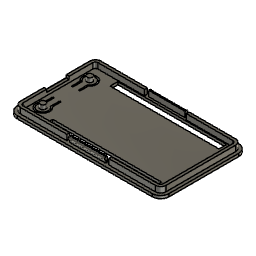
esp32-case (Autodesk Fusion 360 design; units mm, degrees)
Autodesk Fusion 360 part; units mm, degrees
sketch "Sketch3" plane through (0, 0, 0) normal (0, 0, 1) x (1, 0, 0)
  line L0 (0, 13.1652) -> (0, -15.9653) construction
  line L1 (-26.7542, 0) -> (30.5292, 0) construction
  line L2 (23.4, 11.7) -> (-23.4, 11.7)
  line L3 (-23.4, 11.7) -> (-23.4, -11.7)
  line L4 (-23.4, -11.7) -> (23.4, -11.7)
  line L5 (23.4, -11.7) -> (23.4, 11.7)
  line L6 (23.4, 11.7) -> (-23.4, -11.7) construction
  line L7 (-23.4, 11.7) -> (23.4, -11.7) construction
  line L8 (24.2, 14.5) -> (-24.2, 14.5)
  line L9 (-26.2, 12.5) -> (-26.2, -12.5)
  line L10 (-24.2, -14.5) -> (24.2, -14.5)
  line L11 (26.2, -12.5) -> (26.2, 12.5)
  line L12 (26.2, 14.5) -> (-26.2, -14.5) construction
  line L13 (-26.2, 14.5) -> (26.2, -14.5) construction
  arc A0 (-24.2, 14.5) -> (-26.2, 12.5) centre (-24.2, 12.5) ccw
  arc A1 (-26.2, -12.5) -> (-24.2, -14.5) centre (-24.2, -12.5) ccw
  arc A2 (24.2, -14.5) -> (26.2, -12.5) centre (24.2, -12.5) ccw
  arc A3 (26.2, 12.5) -> (24.2, 14.5) centre (24.2, 12.5) ccw
  circle A4 centre (23.4, 11.7) radius 1.1
  line L14 (23.4, 10.6) -> (26.2, 10.6)
  line L15 (22.3, 11.7) -> (22.3, 14.5)
  circle A5 centre (-23.4, 11.7) radius 1.1
  line L16 (-22.3, 11.7) -> (-22.3, 14.5)
  line L17 (-23.4, 10.6) -> (-26.2, 10.6)
  line L18 (23.4, -10.6) -> (26.2, -10.6)
  line L19 (22.3, -11.7) -> (22.3, -14.5)
  circle A6 centre (23.4, -11.7) radius 1.1
  line L20 (-22.3, -11.7) -> (-22.3, -14.5)
  circle A7 centre (-23.4, -11.7) radius 1.1
  line L21 (-23.4, -10.6) -> (-26.2, -10.6)
  line L22 (-24.2, -15.5) -> (24.2, -15.5)
  arc A8 (24.2, -15.5) -> (27.2, -12.5) centre (24.2, -12.5) ccw
  line L23 (27.2, -12.5) -> (27.2, 12.5)
  arc A9 (27.2, 12.5) -> (24.2, 15.5) centre (24.2, 12.5) ccw
  line L24 (24.2, 15.5) -> (-24.2, 15.5)
  arc A10 (-24.2, 15.5) -> (-27.2, 12.5) centre (-24.2, 12.5) ccw
  line L25 (-27.2, 12.5) -> (-27.2, -12.5)
  arc A11 (-27.2, -12.5) -> (-24.2, -15.5) centre (-24.2, -12.5) ccw
  line L26 (-16.7, 14.5) -> (-16.7, 11.7)
  line L27 (-16.7, -14.5) -> (-16.7, -11.7)
  line L28 (-26.2, 0) -> (-27.2, 0)
  line L29 (-27.2, 0) -> (-27.2, 4)
  line L30 (-27.2, 4) -> (-26.2, 4)
  line L31 (-26.2, 4) -> (-26.2, 0)
  line L32 (-27.2, 0) -> (-27.2, -4)
  line L33 (-27.2, -4) -> (-26.2, -4)
  line L34 (-26.2, 0) -> (-27.2, 0)
  dimension "d52" = 46.8
  dimension "d53" = 23.4
  dimension "d54" = 29
  dimension "d55" = 52.4
  dimension "d56" = 2
  dimension "d57" = 2.2
  dimension "d59" = 1
  dimension "d61" = 39
  dimension "d78" = 4
  dimension "d79" = 1
  constraint vertical L0
  constraint horizontal L1
  constraint horizontal L2
  constraint perpendicular L2 L3
  constraint parallel L2 L4
  constraint parallel L3 L5
  constraint coincident L6 origin
  constraint coincident L7 origin
  constraint horizontal L8
  constraint perpendicular L8 L9
  constraint parallel L8 L10
  constraint parallel L9 L11
  constraint coincident L12 origin
  constraint coincident L13 origin
  constraint coincident L13.start L8
  constraint coincident L13.start L9
  constraint tangent L8 A0
  constraint tangent L9 A0
  constraint coincident L12.end L9
  constraint coincident L12.end L10
  constraint tangent L9 A1
  constraint tangent L10 A1
  constraint equal A0 A1
  constraint coincident L13.end L10
  constraint coincident L13.end L11
  constraint tangent L10 A2
  constraint tangent L11 A2
  constraint equal A0 A2
  constraint coincident L12.start L11
  constraint coincident L12.start L8
  constraint tangent L11 A3
  constraint tangent L8 A3
  constraint equal A0 A3
  constraint coincident L2.start L5.end
  constraint coincident A4 L14.start
  constraint coincident L5 L14.start
  constraint coincident L11 L14.end
  constraint tangent A4 L14
  constraint coincident A4 L15.start
  constraint coincident L2 L15.start
  constraint coincident L8 L15.end
  constraint tangent A4 L15
  constraint coincident L1 origin
  constraint coincident L0 origin
  constraint symmetric L0 A4 A5
  constraint symmetric L0 L14.start L17.start
  constraint symmetric L0 L14.end L17.end
  constraint symmetric L0 L15.start L16.start
  constraint symmetric L0 L15.end L16.end
  constraint symmetric L1 A4 A6
  constraint symmetric L1 L14.start L18.start
  constraint symmetric L1 L14.end L18.end
  constraint symmetric L1 L15.start L19.start
  constraint symmetric L1 L15.end L19.end
  constraint symmetric L1 A5 A7
  constraint symmetric L1 L16.start L20.start
  constraint symmetric L1 L16.end L20.end
  constraint symmetric L1 L17.start L21.start
  constraint symmetric L1 L17.end L21.end
  constraint coincident L8 L26.start
  constraint coincident L2 L26.end
  constraint perpendicular L2 L26
  constraint symmetric L1 L26.start L27.start
  constraint symmetric L1 L26.end L27.end
  constraint horizontal L28
  constraint vertical L29
  constraint horizontal L30
  constraint vertical L31
  constraint midpoint L9 L28.start
  constraint symmetric L1 L28.start L31.end
  constraint symmetric L1 L28.end L29.start
  constraint symmetric L1 L29.end L32.end
  constraint symmetric L1 L30.end L33.end
  measures "d52" distance of L3.end L4.end
  measures "d53" distance of L2.end L3.end
  measures "d54" distance of L13.start L12.end
  measures "d55" distance of L13.end L9
  measures "d56" radius of A0
  measures "d57" diameter of A4
  measures "d61" distance of L15 L26
  measures "d78" distance of L28.start L30.end
  measures "d79" distance of L29 L31
extrude "Extrude14" add sketch "Sketch3" along normal blind 1 contours L2 L5 A4 | L2 L5 A4 | L2 L3 L4 L5 A4 A5 A6 A7 | L8 L11 A3 A4 L14 L15 | L5 L11 L14 L18 | L2 L8 L16 L26 | L8 L9 L10 L11 A0 A1 A2 A3 L22 A8 L23 A9 L24 A10 L25 A11 L30 L33 | L4 L5 A6 | L10 L11 A2 L18 L19 A6 | L4 L5 A6 | L2 L3 A5 | L2 L3 A5 | L8 L9 A0 A5 L16 L17 | L3 L9 L17 L21 L31 | L4 L10 L20 L27 | L3 L4 A7 | L3 L4 A7 | L9 L10 A1 L20 A7 L21 | L9 L25 L28 L29 L30 L31 L34 | L9 L25 L28 L32 L33 L34 makes body 1
extrude "Extrude20" add sketch "Sketch3" along normal blind 13.7 contours L8 L9 L10 L11 A0 A1 A2 A3 L22 A8 L23 A9 L24 A10 L25 A11 L30 L33 bodies 1
extrude "Extrude17" add sketch "Sketch3" along normal blind 8.5 contours L8 L11 A3 A4 L14 L15 | L10 L11 A2 L18 L19 A6 | L8 L9 A0 A5 L16 L17 | L9 L10 A1 L20 A7 L21 bodies 1
extrude "Extrude19" add sketch "Sketch3" along normal blind 10 contours L2 L5 A4 | L2 L5 A4 | L4 L5 A6 | L4 L5 A6 | L2 L3 A5 | L2 L3 A5 | L3 L4 A7 | L3 L4 A7 | L9 L25 L28 L29 L30 L31 L34 | L9 L25 L28 L32 L33 L34 bodies 1
chamfer "Chamfer4" distance 1.3 angle 45 2 edges at (-26.7, 4, 10) (-26.7, -4, 10) on bodies 1
sketch "Sketch2" plane through (0, 0, 0) normal (1, 0, 0) x (0, 1, 0)
  line L0 (0, 15.9882) -> (0, -1.7691) construction
  line L1 (14.5, 13.7) -> (15, 13.7)
  line L2 (15, 13.7) -> (15, 11.7)
  line L3 (15, 11.7) -> (14.5, 11.7)
  line L4 (14.5, 11.7) -> (14.5, 13.7)
  line L5 (-12.5, 0) -> (12.5, 0)
  circle A0 centre (15.0004, 13.2) radius 0.5
  circle A1 centre (-15.0004, 13.2) radius 0.5
  line L6 (-14.5, 13.7) -> (-15, 13.7)
  line L7 (-14.5, 11.7) -> (-14.5, 13.7)
  line L8 (-15, 11.7) -> (-14.5, 11.7)
  line L9 (-15, 13.7) -> (-15, 11.7)
  dimension "d26" = 0.5
  dimension "d27" = 2
  dimension "d28" = 14.5
  dimension "d73" = 1
  constraint vertical L0
  constraint horizontal L1
  constraint vertical L2
  constraint horizontal L3
  constraint vertical L4
  constraint coincident origin L0
  constraint coincident L1.end A0
  constraint symmetric L0 L1.start L6.start
  constraint symmetric L0 L1.end L6.end
  constraint symmetric L0 L2.end L8.start
  constraint symmetric L0 L3.end L7.start
  constraint symmetric L0 A0 A1
  measures "d26" distance of L1.start L1.end
  measures "d27" distance of L1.start L3.end
  measures "d28" distance of L0 L4
  measures "d73" diameter of A0
extrude "Extrude18" cut sketch "Sketch2" along normal mid plane 14 contours L1 L4 A0 | L2 L3 L4 A0 | A1 L7 L8 L9 | A1 L6 L7 bodies 1
sketch "Sketch4" plane through (0, 0, 0) normal (0, 0, 1) x (1, 0, 0)
  line L0 (0, 24.6712) -> (0, -25.9096) construction
  line L1 (-37.8993, 0) -> (40.7367, 0) construction
  line L2 (-24.2, -14.5) -> (24.2, -14.5)
  line L3 (26.2, -12.5) -> (26.2, 12.5)
  line L4 (24.2, 14.5) -> (-24.2, 14.5)
  line L5 (-26.2, 12.5) -> (-26.2, -12.5)
  line L6 (-26.2, -14.5) -> (26.2, 14.5) construction
  line L7 (26.2, -14.5) -> (-26.2, 14.5) construction
  arc A0 (-24.2, 14.5) -> (-26.2, 12.5) centre (-24.2, 12.5) ccw
  arc A1 (-26.2, -12.5) -> (-24.2, -14.5) centre (-24.2, -12.5) ccw
  arc A2 (24.2, -14.5) -> (26.2, -12.5) centre (24.2, -12.5) ccw
  arc A3 (26.2, 12.5) -> (24.2, 14.5) centre (24.2, 12.5) ccw
  line L8 (-24.2, -15.5) -> (24.2, -15.5)
  arc A4 (24.2, -15.5) -> (27.2, -12.5) centre (24.2, -12.5) ccw
  line L9 (27.2, -12.5) -> (27.2, 12.5)
  arc A5 (27.2, 12.5) -> (24.2, 15.5) centre (24.2, 12.5) ccw
  line L10 (24.2, 15.5) -> (-24.2, 15.5)
  arc A6 (-24.2, 15.5) -> (-27.2, 12.5) centre (-24.2, 12.5) ccw
  line L11 (-27.2, 12.5) -> (-27.2, -12.5)
  arc A7 (-27.2, -12.5) -> (-24.2, -15.5) centre (-24.2, -12.5) ccw
  line L12 (-26.1, 12.5) -> (-26.1, -12.5)
  arc A8 (-26.1, -12.5) -> (-24.2, -14.4) centre (-24.2, -12.5) ccw
  line L13 (-24.2, -14.4) -> (24.2, -14.4)
  arc A9 (24.2, -14.4) -> (26.1, -12.5) centre (24.2, -12.5) ccw
  line L14 (26.1, -12.5) -> (26.1, 12.5)
  arc A10 (26.1, 12.5) -> (24.2, 14.4) centre (24.2, 12.5) ccw
  line L15 (24.2, 14.4) -> (-24.2, 14.4)
  arc A11 (-24.2, 14.4) -> (-26.1, 12.5) centre (-24.2, 12.5) ccw
  line L16 (-24.2, -13.4) -> (24.2, -13.4)
  arc A12 (24.2, -13.4) -> (25.1, -12.5) centre (24.2, -12.5) ccw
  line L17 (25.1, -12.5) -> (25.1, 12.5)
  arc A13 (25.1, 12.5) -> (24.2, 13.4) centre (24.2, 12.5) ccw
  line L18 (24.2, 13.4) -> (-24.2, 13.4)
  arc A14 (-24.2, 13.4) -> (-25.1, 12.5) centre (-24.2, 12.5) ccw
  line L19 (-25.1, 12.5) -> (-25.1, -12.5)
  arc A15 (-25.1, -12.5) -> (-24.2, -13.4) centre (-24.2, -12.5) ccw
  line L20 (-22.1, 14.4) -> (-26.1, 14.4) construction
  line L21 (-26.1, 14.4) -> (-26.1, 8.4) construction
  line L22 (-26.1, 8.4) -> (-22.1, 8.4) construction
  line L23 (-22.1, 8.4) -> (-22.1, 14.4) construction
  circle A16 centre (-22.1, 8.4) radius 1
  circle A17 centre (-22.1, 8.4) radius 2
  circle A18 centre (-22.1, 8.4) radius 2.5
  line L24 (-23.6, 3.4) -> (-20.6, 3.4)
  line L25 (-20.6, 3.4) -> (-20.6, 13.4)
  line L26 (-20.6, 13.4) -> (-23.6, 13.4)
  line L27 (-23.6, 13.4) -> (-23.6, 3.4)
  line L28 (-23.6, 3.4) -> (-20.6, 13.4) construction
  line L29 (-20.6, 3.4) -> (-23.6, 13.4) construction
  line L30 (-23.1, 13.4) -> (-21.1, 13.4)
  line L31 (-21.1, 13.4) -> (-21.1, 3.4)
  line L32 (-21.1, 3.4) -> (-23.1, 3.4)
  line L33 (-23.1, 3.4) -> (-23.1, 13.4)
  line L34 (-23.1, 13.4) -> (-21.1, 3.4) construction
  line L35 (-21.1, 13.4) -> (-23.1, 3.4) construction
  circle A19 centre (-22.1, -8.4) radius 1
  circle A20 centre (-22.1, -8.4) radius 2
  circle A21 centre (-22.1, -8.4) radius 2.5
  line L36 (-20.6, -3.4) -> (-20.6, -13.4)
  line L37 (-21.1, -13.4) -> (-21.1, -3.4)
  line L38 (-23.1, -3.4) -> (-23.1, -13.4)
  line L39 (-23.6, -13.4) -> (-23.6, -3.4)
  line L40 (-21.1, -3.4) -> (-23.1, -3.4)
  line L41 (-23.6, -3.4) -> (-20.6, -3.4)
  line L42 (-25.1, 0) -> (-26.1, 0)
  line L43 (-26.1, 0) -> (-26.1, -4)
  line L44 (-26.1, -4) -> (-25.1, -4)
  line L45 (-25.1, -4) -> (-25.1, 0)
  line L46 (-26.1, 4) -> (-25.1, 4)
  line L47 (23.4, 11.7) -> (-23.4, 11.7) construction
  line L48 (-23.4, 11.7) -> (-23.4, -11.7) construction
  line L49 (-23.4, -11.7) -> (23.4, -11.7) construction
  line L50 (23.4, -11.7) -> (23.4, 11.7) construction
  line L51 (23.4, 11.7) -> (-23.4, -11.7) construction
  line L52 (-23.4, 11.7) -> (23.4, -11.7) construction
  line L53 (23.4, 13.1) -> (-23.4, 13.1) construction
  line L54 (23.4, 10.3) -> (-23.4, 10.3) construction
  line L55 (22.3, -11.7) -> (22.3, 11.7) construction
  line L56 (22.3, 10.3) -> (-16.7, 10.3)
  line L57 (-16.7, 10.3) -> (-16.7, 13.1)
  line L58 (-16.7, 13.1) -> (22.3, 13.1)
  line L59 (22.3, 13.1) -> (22.3, 10.3)
  line L60 (-16.7, -10.3) -> (-16.7, -13.1)
  line L61 (22.3, -10.3) -> (-16.7, -10.3)
  line L62 (22.3, -13.1) -> (22.3, -10.3)
  line L63 (-16.7, -13.1) -> (22.3, -13.1)
  line L64 (7.5, -15.5) -> (-7.5, -15.5) construction
  line L65 (-7.5, -15.5) -> (-7.5, 15.5) construction
  line L66 (-7.5, 15.5) -> (7.5, 15.5) construction
  line L67 (7.5, 15.5) -> (7.5, -15.5) construction
  line L68 (7.5, -15.5) -> (-7.5, 15.5) construction
  line L69 (-7.5, -15.5) -> (7.5, 15.5) construction
  line L70 (-7.5, 15.5) -> (-6.5, 15.5) construction
  line L71 (-6.5, 15.5) -> (-6.5, -15.5)
  line L72 (-6.5, -15.5) -> (-7.5, -15.5)
  line L73 (-7.5, -15.5) -> (-7.5, 15.5)
  line L74 (7.5, -15.5) -> (7.5, 15.5)
  line L75 (6.5, 15.5) -> (6.5, -15.5)
  point P0 (-22.1, 8.4)
  point P1 (-22.1, 8.4)
  dimension "d95" = 52.4
  dimension "d96" = 2
  dimension "d97" = 1
  dimension "d98" = 29
  dimension "d99" = -0.1
  dimension "d100" = -1.1
  dimension "d101" = 6
  dimension "d102" = 4
  dimension "d103" = 2
  dimension "d104" = 1
  dimension "d105" = 1.5
  dimension "d106" = 3
  dimension "d107" = 10
  dimension "d108" = 2
  dimension "d109" = 10
  dimension "d114" = 4
  dimension "d119" = 46.8
  dimension "d120" = 23.4
  dimension "d121" = 1.4
  dimension "d122" = -1.4
  dimension "d123" = -1.1
  dimension "d124" = 2.8
  dimension "d125" = 39
  dimension "d128" = 15
  dimension "d129" = 31
  dimension "d130" = 1
  dimension "d131" = 31
  constraint horizontal L2
  constraint perpendicular L2 L3
  constraint parallel L2 L4
  constraint parallel L3 L5
  constraint coincident L6 origin
  constraint coincident L7 origin
  constraint coincident L7.end L4
  constraint coincident L7.end L5
  constraint tangent L4 A0
  constraint tangent L5 A0
  constraint coincident L6.start L5
  constraint coincident L6.start L2
  constraint tangent L5 A1
  constraint tangent L2 A1
  constraint equal A0 A1
  constraint coincident L7.start L2
  constraint coincident L7.start L3
  constraint tangent L2 A2
  constraint tangent L3 A2
  constraint equal A0 A2
  constraint coincident L6.end L3
  constraint coincident L6.end L4
  constraint tangent L3 A3
  constraint tangent L4 A3
  constraint equal A0 A3
  constraint horizontal L20
  constraint vertical L21
  constraint horizontal L22
  constraint vertical L23
  constraint coincident L12 L21.end
  constraint coincident L15 L20.start
  constraint coincident P1 P0
  constraint horizontal L24
  constraint perpendicular L24 L25
  constraint parallel L24 L26
  constraint parallel L25 L27
  constraint coincident L28 P1
  constraint coincident L29 P1
  constraint horizontal L30
  constraint perpendicular L30 L31
  constraint parallel L30 L32
  constraint parallel L31 L33
  constraint coincident L34 P1
  constraint coincident L35 P1
  constraint symmetric L1 A16 A19
  constraint symmetric L1 A17 A20
  constraint symmetric L1 A18 A21
  constraint symmetric L1 L24.start L39.end
  constraint symmetric L1 L24.end L36.start
  constraint symmetric L1 L25.end L36.end
  constraint symmetric L1 L26.end L39.start
  constraint symmetric L1 L30.start L38.end
  constraint symmetric L1 L30.end L37.start
  constraint symmetric L1 L31.end L37.end
  constraint symmetric L1 L32.end L38.start
  constraint horizontal L42
  constraint vertical L43
  constraint horizontal L44
  constraint vertical L45
  constraint midpoint L19 L42.start
  constraint perpendicular L0 L1
  constraint coincident origin L1
  constraint symmetric L1 L43.end L46.start
  constraint symmetric L1 L44.end L46.end
  constraint horizontal L47
  constraint perpendicular L47 L48
  constraint parallel L47 L49
  constraint parallel L48 L50
  constraint coincident L51 origin
  constraint coincident L52 origin
  constraint horizontal L56
  constraint vertical L57
  constraint horizontal L58
  constraint vertical L59
  constraint coincident L55 L56.start
  constraint coincident L54 L56.start
  constraint symmetric L1 L56.start L61.start
  constraint symmetric L1 L56.end L60.start
  constraint symmetric L1 L57.end L60.end
  constraint symmetric L1 L58.end L62.start
  constraint horizontal L64
  constraint perpendicular L64 L65
  constraint parallel L64 L66
  constraint parallel L65 L67
  constraint coincident L68 origin
  constraint coincident L69 origin
  constraint horizontal L70
  constraint vertical L71
  constraint horizontal L72
  constraint vertical L73
  constraint symmetric L0 L65.end L66.end
  constraint symmetric L0 L70.end L75.start
  constraint symmetric L0 L71.end L75.end
  constraint symmetric L0 L64.end L64.start
  measures "d95" distance of L3 L5
  measures "d96" radius of A0
  measures "d98" distance of L2 L4
  measures "d101" distance of L20.start P1
  measures "d102" distance of L21.end P1
  measures "d103" diameter of A16
  measures "d104" distance of A16
  measures "d106" distance of L25.end L26.end
  measures "d107" distance of L24.end L25.end
  measures "d108" distance of L31.end L32.end
  measures "d109" distance of L30.end L31.end
  measures "d114" distance of L42.start L44.end
  measures "d119" distance of L48.end L49.end
  measures "d120" distance of L47.end L48.end
  measures "d124" distance of L56.start L58.end
  measures "d125" distance of L55 L57
  measures "d128" distance of L65.end L66.end
  measures "d129" distance of L64.end L65.end
  measures "d130" distance of L65.end L70.end
  measures "d131" distance of L65.end L64.end
extrude "Extrude25" add sketch "Sketch4" along normal blind 1 separate body contours L2 L4 L5 A0 A1 L12 A8 L13 L15 A11 L43 L73 | L2 L4 L5 A0 A1 L8 L10 A6 L11 A7 L73 | L2 L13 L71 L73 | L2 L8 L71 L72 L73 | L2 L13 L71 L75 | L2 L8 L71 L75 | L13 L16 L71 L73 | L12 A8 L13 L16 L19 A15 L44 L73 | L2 L13 L74 L75 | L2 L8 L74 L75 | L13 L16 L71 L75 | L16 L63 L71 L73 | L16 L18 A14 L19 A15 A18 L24 L25 L27 L32 A21 L36 L39 L40 L41 L45 L56 L57 L58 L60 L61 L63 L73 | L2 L3 L4 A2 A3 L13 A9 L14 A10 L15 L74 | L2 L3 L4 A2 A3 L8 A4 L9 A5 L10 L74 | L13 L16 L74 L75 | L16 L63 L71 L75 | L16 A21 L36 L37 | L4 L10 L71 L73 | L4 L15 L71 L73 | L13 A9 L14 A10 L15 L16 A12 L17 A13 L18 L74 | L16 L63 L74 L75 | L12 L19 L42 L43 L44 L45 | L16 A21 L37 L38 | L56 L61 L71 L73 | L4 L10 L71 L75 | L4 L15 L71 L75 | L12 L15 A11 L18 A14 L19 L26 L30 L46 L73 | L15 L18 L71 L73 | L16 A12 L17 A13 L18 L56 L58 L59 L61 L62 L63 L74 | L56 L61 L71 L75 | L12 L19 L42 L46 | L16 A21 L38 L39 | A20 L36 | A20 L36 L37 | L4 L10 L74 L75 | L4 L15 L74 L75 | L15 L18 L71 L75 | L18 L58 L71 L73 | L56 L61 L74 L75 | A19 A20 L37 L38 | L15 L18 L74 L75 | L18 L58 L71 L75 | L18 A18 L25 L26 L31 | A20 L38 L39 | A19 | A19 A20 L37 L38 | A20 A21 L37 L38 | A21 L37 L38 L40 L41 | L18 L58 L74 L75 | L18 A18 L26 L30 L31 L33 | A20 L39 | L18 A18 L26 L27 L33 | A17 L25 L31 | A17 L25 | A16 A17 L31 L33 | A17 L27 L33 | A16 | A16 A17 L31 L33 | A18 L24 L31 L32 L33 | A17 A18 L31 L33 | A17 L27 picked at (-21.9362, -6.0764) picked at (-21.9362, 6.0764) makes body 2
extrude "Extrude24" add sketch "Sketch4" along normal blind 2 contours L12 L19 L42 L43 L44 L45 | L12 L19 L42 L46 bodies 2
extrude "Extrude26" add sketch "Sketch4" along normal blind 3 contours L12 A8 L13 L16 L19 A15 L44 L73 | L13 L16 L71 L75 | L13 A9 L14 A10 L15 L16 A12 L17 A13 L18 L74 | L12 L15 A11 L18 A14 L19 L26 L30 L46 L73 | L15 L18 L71 L75 bodies 2
extrude "Extrude22" add sketch "Sketch4" along normal blind 2.5 contours A19 | A16 bodies 2
sketch "Sketch5" plane through (0, 0, 0) normal (1, 0, 0) x (0, 1, 0)
  line L0 (14.4, 5.4385) -> (14.4, -1.7536) construction
  line L1 (0, 7.3147) -> (0, -3.5673) construction
  circle A0 centre (14.4, 2.5) radius 0.5
  line L2 (13.9, 3.8955) -> (13.9, -1.5855) construction
  line L3 (-1.6674, 0) -> (18.5491, 0) construction
  line L4 (-1.2492, 3) -> (18.4327, 3) construction
  line L5 (13.9, 3) -> (13.4, 3)
  line L6 (13.4, 3) -> (13.4, 1)
  line L7 (13.4, 1) -> (13.9, 1)
  line L8 (13.9, 1) -> (13.9, 3)
  circle A1 centre (-14.4, 2.5) radius 0.5
  line L9 (-13.9, 1) -> (-13.9, 3)
  line L10 (-13.4, 1) -> (-13.9, 1)
  line L11 (-13.4, 3) -> (-13.4, 1)
  line L12 (-13.9, 3) -> (-13.4, 3)
  dimension "d134" = 14.4
  dimension "d135" = 1
  dimension "d136" = 0.5
  dimension "d137" = 2.5
  dimension "d138" = 3
  dimension "d139" = 0.5
  dimension "d140" = 2
  constraint vertical L0
  constraint vertical L1
  constraint coincident origin L1
  constraint parallel L0 L2
  constraint perpendicular L1 L3
  constraint perpendicular L0 L4
  constraint horizontal L5
  constraint vertical L6
  constraint horizontal L7
  constraint vertical L8
  constraint coincident L2 L5.start
  constraint coincident L4 L5.start
  constraint symmetric L1 A0 A1
  constraint symmetric L1 L5.start L9.end
  constraint symmetric L1 L5.end L11.start
  constraint symmetric L1 L6.end L10.start
  constraint symmetric L1 L7.end L9.start
  measures "d134" distance of L0 L1
  measures "d135" diameter of A0
  measures "d136" distance of L0 L2
  measures "d137" distance of A0.centre L3
  measures "d138" distance of L3 L4
  measures "d139" distance of L5.start L5.end
  measures "d140" distance of L5.start L7.end
extrude "Extrude28" cut sketch "Sketch5" along normal mid plane 13 contours L5 L6 L7 L8 | L9 L10 L11 L12 bodies 2
extrude "Extrude27" add sketch "Sketch5" along normal mid plane 13 contours A0 | A1 bodies 2
hidden bodies 1
equation "width_base = 46.8 mm"
equation "width_total = width_base + ( ( offset_base + depth ) * 2 )"
equation "depth = 1 mm"
equation "window_width = 39 mm"
equation "d26 = depth / 2"
equation "d27 = depth * 2"
equation "d28 = height_total / 2 - depth"
equation "height_base = 23.4 mm"
equation "height_total = height_base + ( offset_base + depth ) * 2"
equation "offset_base = 2.8 mm"
equation "d52 = width_base"
equation "d53 = height_base"
equation "d54 = height_base + offset_base * 2"
equation "d55 = width_base + offset_base * 2"
equation "d56 = depth * 2"
equation "d59 = depth"
equation "d61 = window_width"
equation "d62 = depth"
equation "d73 = depth"
equation "d79 = depth"
equation "d95 = width_base + offset_base * 2"
equation "d96 = depth * 2"
equation "d97 = depth"
equation "d98 = height_base + offset_base * 2"
equation "d100 = -depth - 0.1 mm"
equation "d101 = depth + 5 mm"
equation "d102 = depth + 3 mm"
equation "d112 = depth + 1.5 mm"
equation "d117 = depth + 1 mm"
equation "d119 = width_base"
equation "d121 = offset_base / 2"
equation "d122 = -offset_base / 2"
equation "d123 = -depth - 0.1 mm"
equation "d124 = offset_base"
equation "d125 = window_width"
equation "d126 = depth"
equation "d128 = 14 mm + depth"
equation "d129 = height_total"
equation "d130 = depth"
equation "d131 = height_total"
equation "d132 = depth * 3"
equation "d134 = height_base / 2 + offset_base - 0.1 mm"
equation "d135 = depth"
equation "d136 = depth / 2"
equation "d137 = depth * 3 - depth / 2"
equation "d138 = depth * 3"
equation "d139 = depth / 2"
equation "d140 = depth * 2"
